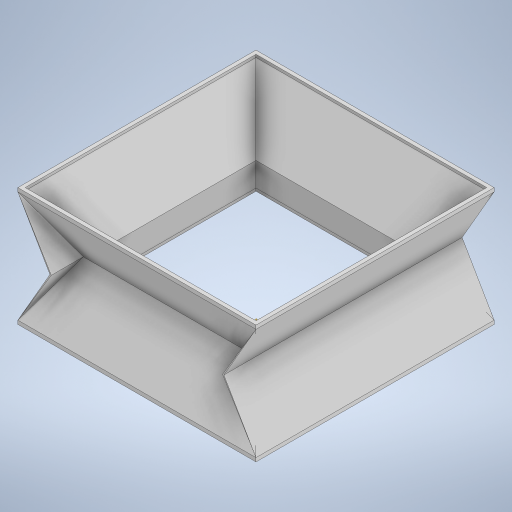
# Autodesk Inventor part: 사각형 OV-PAM 5패턴 층 한개
Saved by Autodesk Inventor 2024 (Build 280153000, 153)
## iProperties
Created: 2023-06-16
Part Number: 사각형 OV-PAM 5패턴 층 한개
Material: 일반
Document SubType Name: Modeling
Designer: jsw
Density: 1 g/cm^3
Appearance: 기본값
Author: jsw
Autodesk Inventor part; units mm, degrees
sketch "스케치1" plane through (0, 0, 0) normal (0, 1, 0) x (-1, 0, 0)
  line L0 (0, 0) -> (-51.451, 0)
  line L1 (-51.451, 0) -> (-51.451, -51.451)
  line L2 (-51.451, -51.451) -> (0, -51.451)
  line L3 (0, -51.451) -> (0, 0)
  line L4 (-0.8, -0.8) -> (-50.651, -0.8)
  line L5 (-50.651, -0.8) -> (-50.651, -50.651)
  line L6 (-50.651, -50.651) -> (-0.8, -50.651)
  line L7 (-0.8, -50.651) -> (-0.8, -0.8)
  dimension "d32" = 70.5
  dimension "d33" = 0.8
  dimension "d34" = 0.8
  dimension "d35" = 0.8
  dimension "d36" = 0.8
  constraints: 16 end point, 4 parallel, 3 perpendicular, 2 horizontal
  measures "d32" distance of L4.end L6.end
  measures "d33" distance between parallel lines of L6 L2
  measures "d34" distance between parallel lines of L7 L3
  measures "d35" distance between parallel lines of L0 L4
  measures "d36" distance between parallel lines of L1 L5
extrude "돌출1" add sketch "스케치1" along normal blind 12 contours L3 L2 L1 L0 | L7 L6 L5 L4
ref_plane "작업 평면1" through (0, 0, 0) normal (0, 0.5, 0.8660254) x (1, 0, 0)
sketch "스케치2" plane through (0, 0, 0) normal (0, 0, 1) x (1, 0, 0)
  line L0 (51.451, 0) -> (0, 0) projected
  line L1 (0, 0) -> (7.2255, 12)
  line L2 (51.451, 12) -> (0, 12) projected
  line L3 (51.451, 0) -> (44.2255, 12)
  line L4 (7.2255, 12) -> (44.2255, 12)
  line L5 (51.451, 0) -> (0, 0)
  point P0 (44.2255, 12)
  point P1 (25.7255, 12)
  dimension "d27" = 37
  dimension "d28" = 18.5
  constraints: 8 end point, 2 collinear, 1 midpoint, 1 point on line
  measures "d27" distance of L1.end L3.end
  measures "d28" distance of L1.end point (25.726, 12)
extrude "돌출2" cut sketch "스케치2" against normal up to surface surface through (0, 0, 0) normal (0, 0.5, 0.8660254)
ref_plane "작업 평면2" through (51.451, 0, 0) normal (0.8660254, 0.5, 0) x (0, 0, -1)
sketch "스케치3" plane through (51.451, 0, -51.451) normal (1, 0, 0) x (0, 0, -1)
  line L0 (0, 12) -> (-51.451, 12) projected
  line L1 (-51.451, 12) -> (0, 12)
  line L2 (0, 12) -> (0, 0)
  line L3 (0, 0) -> (-51.451, 0)
  line L4 (-51.451, 0) -> (-51.451, 12)
  line L5 (-51.451, 0) -> (-58.3792, 12)
  line L6 (-58.3792, 12) -> (-51.451, 12)
  line L7 (0, 0) -> (6.9282, 12)
  line L8 (6.9282, 12) -> (0, 12)
  point P0 (-51.451, 0)
  point P1 (0, 12)
  dimension "d11" = 120
  dimension "d12" = 120
  constraints: 16 end point, 2 collinear, 2 parallel, 1 horizontal, 1 perpendicular, 1 point on line
  measures "d11" angle of L5 L3
  measures "d12" angle of L3 L7
extrude "돌출3" cut sketch "스케치3" along normal up to surface surface through (51.451, 0, 0) normal (0.8660254, 0.5, 0)
pattern_circular "원형 패턴1" count 2 over 360 about axis through (25.7255, 0, -25.7255) along (0, -1, 0) of "돌출3", "돌출2"
mirror "미러1" about plane through (25.7255, 12, -25.7255) normal (0, 1, 0) of "돌출3", "돌출2", "돌출1", "원형 패턴1"
sketch "스케치6" plane through (0, 24, -51.451) normal (0, 1, 0) x (1, 0, 0)
  line L0 (51.451, -51.451) -> (51.451, 0) projected
  line L1 (51.451, 0) -> (0, 0) projected
  line L2 (0, 0) -> (0, -51.451) projected
  line L3 (0, -51.451) -> (51.451, -51.451) projected
extrude "돌출6" add sketch "스케치6" along normal blind 0.8
ref_plane "작업 평면4" through (0, 12, 0) normal (0, -1, 0) x (1, 0, 0)
mirror "미러3" about plane through (0, 12, 0) normal (0, -1, 0) of "돌출6"
shell "쉘4" thickness 0.8 removed faces 2 at (34.3007, 24.8, -17.1503) at (34.3007, -0.8, -17.1503)
equation "\"d28\" = 0.5 * d27"
